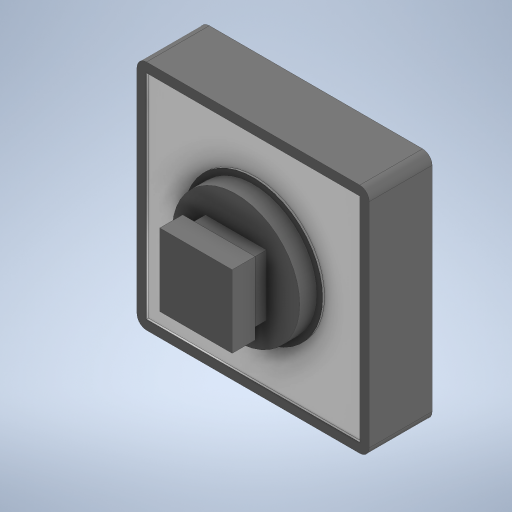
# Autodesk Inventor part: 텍트 스위치
Saved by Autodesk Inventor 2023 (Build 270158000, 158)
## iProperties
Created: 2022-06-24
Part Number: 텍트 스위치
Material: 일반
Document SubType Name: Modeling
Designer: user
Density: 1 g/cm^3
Appearance: 기본값
Author: user
Autodesk Inventor part; units mm, degrees
ref_plane "YZ Plane" through (0, 0, 0) normal (1, 0, 0) x (0, 1, 0)
ref_plane "XZ Plane" through (0, 0, 0) normal (0, 1, 0) x (-1, 0, 0)
ref_plane "XY Plane" through (0, 0, 0) normal (0, 0, 1) x (1, 0, 0)
sketch "스케치1" plane through (0, 0, 0) normal (0, 0, 1) x (1, 0, 0)
  line L0 (-6.1, 6.1) -> (6.1, 6.1)
  line L1 (6.1, 6.1) -> (6.1, -6.1)
  line L2 (6.1, -6.1) -> (-6.1, -6.1)
  line L3 (-6.1, -6.1) -> (-6.1, 6.1)
  line L4 (-6.1, 6.1) -> (6.1, -6.1) construction
  line L5 (6.1, 6.1) -> (-6.1, -6.1) construction
  circle A0 centre (0, 0) radius 3.35
  line L6 (-1.6, 1.6) -> (1.6, 1.6)
  line L7 (1.6, 1.6) -> (1.6, -1.6)
  line L8 (1.6, -1.6) -> (-1.6, -1.6)
  line L9 (-1.6, -1.6) -> (-1.6, 1.6)
  line L10 (-1.6, 1.6) -> (1.6, -1.6) construction
  line L11 (1.6, 1.6) -> (-1.6, -1.6) construction
  line L12 (-1.9, 1.9) -> (1.9, 1.9)
  line L13 (1.9, 1.9) -> (1.9, -1.9)
  line L14 (1.9, -1.9) -> (-1.9, -1.9)
  line L15 (-1.9, -1.9) -> (-1.9, 1.9)
  line L16 (-1.9, 1.9) -> (1.9, -1.9) construction
  line L17 (1.9, 1.9) -> (-1.9, -1.9) construction
  point P0 (0, 0)
  dimension "d0" = 12.2
  dimension "d1" = 12.2
  dimension "d2" = 6.7
  dimension "d3" = 3.2
  dimension "d4" = 3.2
  dimension "d5" = 3.8
  dimension "d6" = 3.8
  constraints: 36 end point, 6 midpoint, 6 parallel, 3 horizontal, 3 perpendicular, 1 centre point, 1 coincident
  measures "d0" distance of L1.end L2.end
  measures "d1" distance of L0.end L1.end
  measures "d2" diameter of A0
  measures "d3" distance of L7.end L8.end
  measures "d4" distance of L6.end L7.end
  measures "d5" distance of L13.end L14.end
  measures "d6" distance of L12.end L13.end
extrude "돌출1" add sketch "스케치1" against normal blind 3.3 contours L0 L1 L2 L3 | A0 | L6 L7 L8 L9 | L12 L13 L14 L15
extrude "돌출2" add sketch "스케치1" along normal blind 0.9 contours A0 | L6 L7 L8 L9 | L12 L13 L14 L15
extrude "돌출3" add sketch "스케치1" along normal blind 3 contours L6 L7 L8 L9 | L12 L13 L14 L15
sketch "스케치2" plane through (0, 0, 0.9) normal (0, 0, 1) x (1, 0, 0)
  line L0 (-1.6, -1.6) -> (1.6, -1.6)
  line L1 (1.6, -1.6) -> (1.6, 1.6)
  line L2 (1.6, 1.6) -> (-1.6, 1.6)
  line L3 (-1.6, 1.6) -> (-1.6, -1.6)
  line L4 (-1.6, -1.6) -> (1.6, 1.6) construction
  line L5 (1.6, -1.6) -> (-1.6, 1.6) construction
  line L6 (-1.9, -1.9) -> (1.9, -1.9) projected
  line L7 (1.9, -1.9) -> (1.9, 1.9) projected
  line L8 (1.9, 1.9) -> (-1.9, 1.9) projected
  line L9 (-1.9, 1.9) -> (-1.9, -1.9) projected
  point P0 (0, 0)
  dimension "d13" = 3.2
  dimension "d14" = 3.2
  constraints: 12 end point, 2 midpoint, 2 parallel, 1 horizontal, 1 perpendicular
  measures "d13" distance of L2.end L1.end
  measures "d14" distance of L1.end L0.end
extrude "돌출4" cut sketch "스케치2" along normal blind 0.9
fillet "모깎기1" radius 0.5 4 edges at (6.1, 6.1, -1.65) (6.1, -6.1, -1.65) (-6.1, -6.1, -1.65) (-6.1, 6.1, -1.65)
sketch "스케치3" plane through (0, 0, 0) normal (0, 0, 1) x (1, 0, 0)
  circle A0 centre (0, 0) radius 3.35 projected
  arc A1 (-5.6, 6.1) -> (-6.1, 5.6) centre (-5.6, 5.6) ccw projected
  line L0 (-6.1, 5.6) -> (-6.1, -5.6) projected
  arc A2 (-6.1, -5.6) -> (-5.6, -6.1) centre (-5.6, -5.6) ccw projected
  line L1 (-5.6, -6.1) -> (5.6, -6.1) projected
  arc A3 (5.6, -6.1) -> (6.1, -5.6) centre (5.6, -5.6) ccw projected
  line L2 (6.1, -5.6) -> (6.1, 5.6) projected
  arc A4 (6.1, 5.6) -> (5.6, 6.1) centre (5.6, 5.6) ccw projected
  line L3 (5.6, 6.1) -> (-5.6, 6.1) projected
  line L4 (-5.6, 5.6) -> (-5.6, -5.6)
  line L5 (-5.6, -5.6) -> (5.6, -5.6)
  line L6 (5.6, -5.6) -> (5.6, 5.6)
  line L7 (5.6, 5.6) -> (-5.6, 5.6)
  circle A5 centre (0, 0) radius 3.65
  point P0 (0, 0)
  dimension "d18" = 0.5
  dimension "d19" = 0.3
  constraints: 8 end point, 1 centre point, 3 other
  measures "d18" distance between parallel lines of L3 L7
  measures "d19" radial gap between concentric circles of A0 A5
extrude "돌출5" cut sketch "스케치3" against normal blind 0.1 contours L7 L6 L5 L4
